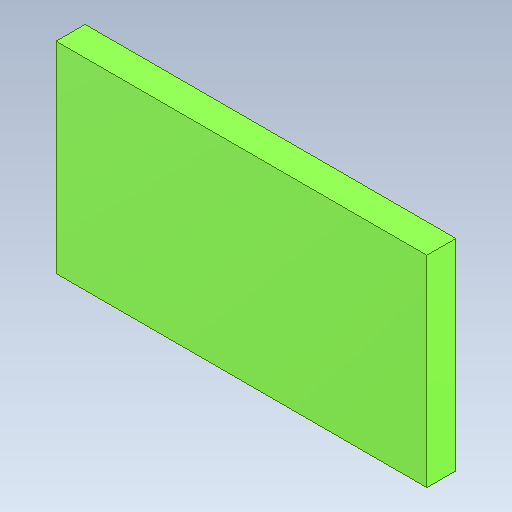
# Autodesk Inventor part: _SWITCH_SPDT_4_7
Saved by Autodesk Inventor 2021 (Build 250183000, 183)
## iProperties
Created: 2020-11-03
Part Number: _SWITCH_SPDT_4_7
Material: Generic
Document SubType Name: Modeling
Designer: faiya
Density: 1 g/cm^3
Appearance: _SWITCH_SPDT_4_7, _SWITCH_SPDT_4_7
Author: faiya
Autodesk Inventor part; units mm, degrees
ref_plane "YZ Plane" through (0, 0, 0) normal (1, 0, 0) x (0, 1, 0)
ref_plane "XZ Plane" through (0, 0, 0) normal (0, 1, 0) x (-1, 0, 0)
ref_plane "XY Plane" through (0, 0, 0) normal (0, 0, 1) x (1, 0, 0)
sketch "_SWITCH_SPDT_4_7, _SWITCH_SPDT_4_7_50" plane through (0, 0, 0) normal (0, 0, 1) x (1, 0, 0)
  line L0 (-6.4135, 3.4635) -> (6.35, 3.4635)
  line L1 (6.35, 3.4635) -> (6.35, -3.4635)
  line L2 (6.35, -3.4635) -> (-6.4135, -3.4635)
  line L3 (-6.4135, -3.4635) -> (-6.4135, 3.4635)
  constraints: 8 end point
extrude "Extrusion1" add sketch "_SWITCH_SPDT_4_7, _SWITCH_SPDT_4_7_50" along normal blind 1
body "Solid1"
